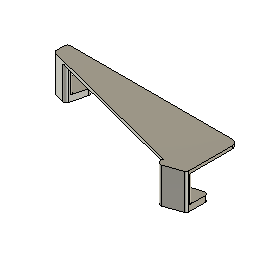
Caliper Hanging Bracket (Autodesk Fusion 360 design; units mm, degrees)
Autodesk Fusion 360 part; units mm, degrees
sketch "Sketch1" plane through (0, 0, 0) normal (0, 0, 1) x (1, 0, 0) in component "Caliper Hanging Bracket"
  line L0 (-49.4372, 12.7953) -> (0, 0)
  line L1 (8.1454, 2.4216) -> (0, 0)
  line L2 (-49.4372, 12.7953) -> (-49.4372, 17.3382)
  line L3 (-49.4372, 17.3382) -> (8.1454, 17.3382)
  line L4 (8.1454, 17.3382) -> (8.1454, 2.4216)
  line L5 (0, 0) -> (0.8806, -2.495)
  line L6 (0.8806, -2.495) -> (8.1454, 0.0691)
  line L7 (8.1454, 0.0691) -> (8.1454, 2.4216)
  line L8 (-49.4372, 12.7953) -> (-49.4372, 15.3629)
  line L9 (-49.4372, 15.3629) -> (-43.7781, 13.8982)
  line L10 (-43.7781, 13.8982) -> (-44.4009, 11.4918)
  dimension "d17" = 4.5429
  dimension "d18" = 57.5826
  dimension "d19" = 5.8456
  dimension "d20" = 51.0662
  dimension "d23" = 7.704
  dimension "d24" = 2.6458
  dimension "d25" = 8.4977
  dimension "d26" = 2.4857
  constraint vertical L2
  constraint horizontal L3
  constraint vertical L4
  constraint vertical L7
  constraint perpendicular L5 L6
  constraint coincident L0 L10.end
  constraint perpendicular L0 L10
  constraint collinear L2 L8
  constraint parallel L0 L9
  constraint coincident L0.end L1.end
  measures "d17" distance of L0.start L2.end
  measures "d18" distance of L2.end L3.end
  measures "d19" distance of L8.end L9.end
  measures "d20" distance of L0.start L0.end
  measures "d23" distance of L5.end L6.end
  measures "d24" distance of L0.end L5.end
  measures "d25" distance of L1.start L0.end
  measures "d26" distance of L9.end L10.end
extrude "Extrude1" add sketch "Sketch1" against normal blind 1 contours L0 L1 L2 L3 L4 L9 L10 makes body 1 in component "Caliper Hanging Bracket"
extrude "Extrude2" add sketch "Sketch1" against normal blind 12 contours L0 L2 L8 L9 L10 | L1 L5 L6 L7 bodies 1 in component "Caliper Hanging Bracket"
ref_plane "WorkPlane1" through (-46.6077, 13.4273, -10) normal (0, 0, -1) x (-1, 0, 0) in component "Caliper Hanging Bracket"
split "Split1" by plane through (-46.6077, 13.4273, -10) normal (0, 0, -1) bodies 1 makes body 2 at (3.0087, -0.8086, -12) makes body 3 at (-47.5509, 14.0188, -12) in component "Caliper Hanging Bracket"
move_face "OffsetFaces1" offset 5 2 faces at (-47.5509, 14.8746, -10.6667) (5.4303, 1.6144, -10.6667) on bodies 2 3 in component "Caliper Hanging Bracket"
combine "Combine1" operation add target body 1 tool bodies 2 3 in component "Caliper Hanging Bracket"
fillet "Fillet1" radius 1 13 edges at (8.1454, 7.6379, -11) (-49.4372, 17.3382, -0.5) (-49.4372, 20.5276, -11) (-49.4372, 15.3629, -5.5) (-49.4372, 12.7953, -6) (-44.4009, 11.4918, -6.5) (-43.7781, 13.8982, -5.5) (8.1454, 0.0691, -6) (8.1454, 2.4216, -5.5) (0.8806, -2.495, -6) (-1.6662, 4.7209, -11) (0, 0, -5.5) (-42.5253, 18.7387, -11) on bodies 1 in component "Caliper Hanging Bracket"
fillet "Fillet2" radius 2 1 edges at (8.1454, 17.3382, -0.5) on bodies 1 in component "Caliper Hanging Bracket"
component "Caliper Hanging Bracket" placed x (1, 0, 0) y (0, 1, 0) z (0, 0, 1) at (0, 0, 0)
named bodies: "Caliper Hanging Bracket"
